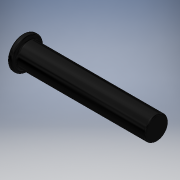
# Autodesk Inventor part: Handle bars handles
Saved by Autodesk Inventor 2018 (Build 220112000, 112)
## iProperties
Created: 2018-08-14
Part Number: Handle bars handles
Material: Generic
Document SubType Name: Modeling
Designer: ruben
Density: 1 g/cm^3
Appearance: Glossy - Black
Author: ruben
Autodesk Inventor part; units mm, degrees
ref_plane "YZ Plane" through (0, 0, 0) normal (1, 0, 0) x (0, 1, 0)
ref_plane "XZ Plane" through (0, 0, 0) normal (0, 1, 0) x (-1, 0, 0)
ref_plane "XY Plane" through (0, 0, 0) normal (0, 0, 1) x (1, 0, 0)
sketch "Sketch1" plane through (0, 0, 0) normal (0, 1, 0) x (-1, 0, 0)
  line L0 (3.8, 0) -> (-22.8, 0) projected
  line L1 (0, -147.7698) -> (0, 222.7404) projected
  line L2 (-11, -80) -> (-19, -80)
  line L3 (-19, -80) -> (-19, -74)
  line L4 (-19, -74) -> (-14, -74)
  line L5 (-14, -74) -> (-14, 80)
  line L6 (-14, 80) -> (0, 80)
  line L7 (-11, -94.8398) -> (-11, 169.8104) construction
  line L8 (-11, -80) -> (-11, 76)
  line L9 (-11, 76) -> (0, 76)
  dimension "d0" = 38
  dimension "d1" = 28
  dimension "d3" = 22
  dimension "d4" = 160
  dimension "d5" = 6
  dimension "d7" = 4
  constraints: 16 end point, 6 perpendicular, 3 point on line, 1 collinear, 1 parallel, 1 other
  measures "d0" diameter of L3 L1
  measures "d1" diameter of L5 L1
  measures "d3" diameter of L7 L1
  measures "d4" distance between parallel lines of L6 L2
  measures "d5" distance between parallel lines of L4 L2
  measures "d7" distance between parallel lines of L6 L9
revolve "Revolution1" add sketch "Sketch1" angle 360 about axis through (0, 0, -10) along (0, 0, 1) contours L8 L2 L3 L4 L5 L0 | L0 L5 L6 L1 L9 L8
fillet "Fillet1" radius 2 4 edges at (-19, 0, -74) (-14, 0, -74) (-14, 0, 80) (-19, 0, -80)
body "Solid1"
